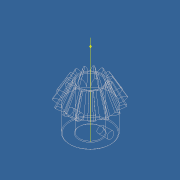
# Autodesk Inventor part: Bevel Gear2
Saved by Autodesk Inventor 2012 SP2 (Build 160219200, 219)
## iProperties
Created: 2012-07-24
Part Number: Bevel Gear2
Material: Steel, Mild
Document SubType Name: Modeling
Designer: bruno.silveira
Categories: <?xml version="1.0" encoding="UTF-16"?> <MemberInstance><Categories><FamilyTemplate><FamilyTemplateParameter ValueType="xs:double" Id="1" ObjectReferenceKey="da_z" ObjectType="kUserParameterObject"/><FamilyTemplateParameter ValueType="xs:double" Id="2" ObjectReferenceKey="da_b" ObjectType="kUserParameterObject"/><FamilyTemplateParameter ValueType="xs:double" Id="3" ObjectReferenceKey="da_beta" ObjectType="kUserParameterObject"/><FamilyTemplateParameter ValueType="xs:double" Id="4" ObjectReferenceKey="da_dae" ObjectType="kUserParameterObject"/><FamilyTemplateParameter ValueType="xs:double" Id="5" ObjectReferenceKey="da_ve" ObjectType="kUserParameterObject"/><FamilyTemplateParameter ValueType="xs:double" Id="6" ObjectReferenceKey="da_omega" ObjectType="kUserParameterObject"/><FamilyTemplateParameter ValueType="xs:string" Id="7" ObjectReferenceKey="EAIAABAAAAAAHwAAAAAAAIAAAAAAAAAA" ObjectType="83914240" SubObjectId="SurfaceGeometry"/></FamilyTemplate><ParamToTemplateMap><ParamToTemplate CategoryParameter="//CategoryParameter[@InternalName='046C89C9-8512-4d59-83FE-43B91F4F132A']" TemplateParameter="1"/><ParamToTemplate CategoryParameter="//CategoryParameter[@InternalName='2552DF32-E462-4b46-AEBF-C6C7768E72AC']" TemplateParameter="2"/><ParamToTemplate CategoryParameter="//CategoryParameter[@InternalName='C9EE641D-15FC-4fae-A226-E94C4372FDD7']" TemplateParameter="3"/><ParamToTemplate><ParamToTemplate CategoryParameter="//CategoryParameter[@InternalName='00B6519A-459B-49c7-AD84-2E56D39A5744']" ConstantValue="-0.000000"/></ParamToTemplate><ParamToTemplate><ParamToTemplate CategoryParameter="//CategoryParameter[@InternalName='04B31F0E-C7A6-4894-AA32-9629BEFACF47']" ConstantValue="1.000000"/></ParamToTemplate><ParamToTemplate><ParamToTemplate CategoryParameter="//CategoryParameter[@InternalName='43CBEC2E-7847-49e7-A936-2F7889FCB2D9']" ConstantValue="0.200000"/></ParamToTemplate><ParamToTemplate><ParamToTemplate CategoryParameter="//CategoryParameter[@InternalName='B1EFC894-105D-4ebd-86BF-FA20ED196853']" ConstantValue="0.300000"/></ParamToTemplate><ParamToTemplate><ParamToTemplate CategoryParameter="//CategoryParameter[@InternalName='51175063-3D10-4879-93E8-6246FE8B403D']" ConstantValue="2060000000.000000"/></ParamToTemplate><ParamToTemplate><ParamToTemplate CategoryParameter="//CategoryParameter[@InternalName='A3A52E27-4454-46a9-B0BD-C932399B70AF']" ConstantValue="0.300000"/></ParamToTemplate><ParamToTemplate CategoryParameter="//CategoryParameter[@InternalName='2A200944-5A8C-41ca-B96E-8520D2E510F1']" TemplateParameter="4"/><ParamToTemplate><ParamToTemplate CategoryParameter="//CategoryParameter[@InternalName='1A637F62-92C8-44bc-B81F-10802510B579']" ConstantValue="1.516492"/></ParamToTemplate><ParamToTemplate CategoryParameter="//CategoryParameter[@InternalName='B52DD4BE-6863-48fb-BF58-89EF6F9EC65C']" TemplateParameter="5"/><ParamToTemplate><ParamToTemplate CategoryParameter="//CategoryParameter[@InternalName='3956BFF2-84D2-457d-93C2-9B0613DEBA67']" ConstantValue="1.315343"/></ParamToTemplate><ParamToTemplate CategoryParameter="//CategoryParameter[@InternalName='739CFA02-461B-4bf8-8049-181FCAD8B28F']" TemplateParameter="6"/><ParamToTemplate><ParamToTemplate CategoryParameter="//CategoryParameter[@InternalName='A27E999F-E2CE-4481-8A2A-EBF499C4C3C5']" ConstantValue="-0.000000"/></ParamToTemplate><ParamToTemplate><ParamToTemplate CategoryParameter="//CategoryParameter[@InternalName='9E1B4470-B2D3-4ff1-B813-535BB4CDF51A']" ConstantValue="3520000.000000"/></ParamToTemplate><ParamToTemplate><ParamToTemplate CategoryParameter="//CategoryParameter[@InternalName='F8452263-BFF6-458c-9FB1-07C4B99E95CD']" ConstantValue="11400000.000000"/></ParamToTemplate><ParamToTemplate><ParamToTemplate CategoryParameter="//CategoryParameter[@InternalName='3E3BB259-FD49-497f-8171-6EBC954A3479']" ConstantValue="2.000000"/></ParamToTemplate><ParamToTemplate CategoryParameter="//CategoryParameter[@InternalName='27C3BAF2-7550-4e4b-AE2C-0DB134B7D9B7']" TemplateParameter="7"/></ParamToTemplateMap><Category DisplayName="Gear" InternalName="DC85795E-93AB-48d5-8EEE-5A27447B64BD" Mnemonic="Gear"><CategoryParameter DisplayName="z" InternalName="046C89C9-8512-4d59-83FE-43B91F4F132A" Mnemonic="z"/><CategoryParameter DisplayName="b" InternalName="2552DF32-E462-4b46-AEBF-C6C7768E72AC" Mnemonic="b"/><CategoryParameter DisplayName="||b|" InternalName="C9EE641D-15FC-4fae-A226-E94C4372FDD7" Mnemonic="beta"/><CategoryParameter DisplayName="x" InternalName="00B6519A-459B-49c7-AD84-2E56D39A5744" Mnemonic="x"/><CategoryParameter DisplayName="a*" InternalName="04B31F0E-C7A6-4894-AA32-9629BEFACF47" Mnemonic="a"/><CategoryParameter DisplayName="c*" InternalName="43CBEC2E-7847-49e7-A936-2F7889FCB2D9" Mnemonic="c"/><CategoryParameter DisplayName="r|.f|*" InternalName="B1EFC894-105D-4ebd-86BF-FA20ED196853" Mnemonic="rf"/><CategoryParameter DisplayName="E" InternalName="51175063-3D10-4879-93E8-6246FE8B403D" Mnemonic="E"/><CategoryParameter DisplayName="||m|" InternalName="A3A52E27-4454-46a9-B0BD-C932399B70AF" Mnemonic="mi"/><Category DisplayName="BevelGear" InternalName="0C98F69A-0C2B-4791-B2FE-7691BB227E77" Mnemonic="BevelGear"><CategoryParameter DisplayName="d|.ae|" InternalName="2A200944-5A8C-41ca-B96E-8520D2E510F1" Mnemonic="dae"/><CategoryParameter DisplayName="d|.ai|" InternalName="1A637F62-92C8-44bc-B81F-10802510B579" Mnemonic="dai"/><CategoryParameter DisplayName="A|.e|" InternalName="B52DD4BE-6863-48fb-BF58-89EF6F9EC65C" Mnemonic="ve"/><CategoryParameter DisplayName="A|.i|" InternalName="3956BFF2-84D2-457d-93C2-9B0613DEBA67" Mnemonic="vi"/><CategoryParameter DisplayName="||S|" InternalName="739CFA02-461B-4bf8-8049-181FCAD8B28F" Mnemonic="omega"/><CategoryParameter DisplayName="x|.t|" InternalName="A27E999F-E2CE-4481-8A2A-EBF499C4C3C5" Mnemonic="xt"/><CategoryParameter DisplayName="||s||.Flim|" InternalName="9E1B4470-B2D3-4ff1-B813-535BB4CDF51A" Mnemonic="sFlim"/><CategoryParameter DisplayName="||s||.Hlim|" InternalName="F8452263-BFF6-458c-9FB1-07C4B99E95CD" Mnemonic="sHlim"/><CategoryParameter DisplayName="type" InternalName="3E3BB259-FD49-497f-8171-6EBC954A3479" Mnemonic="type"/><CategoryParameter DisplayName="PitchDiameter" InternalName="27C3BAF2-7550-4e4b-AE2C-0DB134B7D9B7" Mnemonic="IDS_PITCHDIAM"/></Category></Category></Categories></MemberInstance>
Mass: 60.9118 g
Surface Area: 34.3074 cm^2
Volume: 7.7496 cm^3
Density: 7.86 g/cm^3
CustomPartVersion: 1
Author: bruno.silveira
Autodesk Inventor part; units mm, degrees
ref_plane "Mesh Plane2" through (0, 0, 0) normal (0.9781476, 0.2079117, 0) x (0, 0, 1)
sketch "Teeth Body Sketch" plane through (0, 0, 0) normal (1, 0, 0) x (0, 1, 0)
  line L0 (0, 0) -> (9.640031, -23.304984) construction
  line L1 (9.640031, -23.304984) -> (12.585483, -21.832259)
  line L2 (12.585483, -21.832259) -> (0, 0) construction
  line L3 (11.25, -22.5) -> (0, 0) construction
  line L4 (5.807895, -14.040713) -> (7.582462, -13.153429)
  line L5 (9.640031, -23.304984) -> (5.807895, -14.040713)
  line L6 (12.585483, -21.832259) -> (7.582462, -13.153429)
  line L7 (0, -39.386751) -> (0, 6.564458)
  line L8 (0, -22.5) -> (12.585483, -22.5) construction
  dimension "d0" = 22.5
  dimension "d1" = 19.28006
  dimension "d2" = 25.17097
  dimension "d3" = 10
  dimension "d4" = 21.83226
  constraints: 16 end point, 4 point on line, 3 perpendicular, 2 collinear, 1 horizontal alignment, 1 vertical alignment
  measures "d0" diameter of L3.start L7
  measures "d1" diameter of L0.end L7
  measures "d2" diameter of L1.end L7
  measures "d3" distance between parallel lines of L1 L4
  measures "d4" vertical distance of L1.end L0.start
revolve "Teeth Body" add sketch "Teeth Body Sketch" angle 360 about axis through (0, 0, 0) along (0, 0, 1)
ref_plane "Tooth Plane" through (0, 11.25, -22.5) normal (0, -0.4472136, 0.8944272) x (1, 0, 0)
sketch "Start Sketch" plane through (0, 11.25, -22.5) normal (0, -0.4472136, 0.8944272) x (1, 0, 0)
  line L0 (0, -23.505131) -> (0, 10.644758)
  arc A0 (-0.686149, -2.195174) -> (-3.356057, 2.102319) centre (-5.477944, -2.194063) ccw
  arc A1 (3.356057, 2.102319) -> (0.686149, -2.195174) centre (5.477944, -2.194063) ccw
  line L1 (-0.686149, -2.195174) -> (0.686149, -2.195174)
  arc A2 (3.356057, 2.102319) -> (-3.356057, 2.102319) centre (0, -12.577882) ccw
  dimension "d7" = 4.7918
  dimension "d8" = 5.47794
  dimension "d9" = 10.38382
  dimension "d57" = 15.05893
  dimension "d58" = 10.38271
  constraints: 6 point on circle, 3 centre point, 3 symmetric about line, 2 end point, 1 coincident, 1 perpendicular, 1 other
  measures "d7" radius of A0
  measures "d8" horizontal distance of point (0, -12.578) A0.centre
  measures "d9" vertical distance of point (0, -12.578) A0.centre
  measures "d57" radius of A2
  measures "d58" distance from line of A2.centre L1
sketch "End Sketch" plane through (0, 6.704228, -13.408455) normal (0, -0.4472136, 0.8944272) x (1, 0, 0)
  line L0 (0, -15.358918) -> (0, 6.982715)
  arc A0 (-0.409584, -1.29779) -> (-2.003336, 1.267518) centre (-3.269956, -1.297127) ccw
  arc A1 (2.003336, 1.267518) -> (0.409584, -1.29779) centre (3.269956, -1.297127) ccw
  line L1 (-0.409584, -1.29779) -> (0.409584, -1.29779)
  arc A2 (2.003336, 1.267518) -> (-2.003336, 1.267518) centre (0, -7.495554) ccw
  dimension "d12" = 2.86037
  dimension "d15" = 3.26996
  dimension "d16" = 6.19843
  dimension "d59" = 8.98915
  dimension "d60" = 6.19776
  constraints: 6 point on circle, 3 centre point, 3 symmetric about line, 2 end point, 1 coincident, 1 other
  measures "d12" radius of A0
  measures "d15" horizontal distance of A0.centre point (0, -7.496)
  measures "d16" vertical distance of A0.centre point (0, -7.496)
  measures "d59" radius of A2
  measures "d60" distance from line of A2.centre L1
loft "Loft" cut profiles "Start Sketch", "End Sketch"
pattern_circular "Circular Pattern" count 15 over 360 about axis through (0, 0, 0) along (0, 0, 1) of "Loft"
ref_plane "End Plane" through (0, 6.704228, -13.408455) normal (0, -0.4472136, 0.8944272) x (1, 0, 0)
sketch3d "3D Sketch Right"
ref_plane "End Plane Right" through (-2.675041, 6.147424, -13.408455) normal (0.1784419, -0.4100713, 0.8944272) x (0.9169474, 0.3990081, 0)
sketch "End Sketch Right" plane through (-2.675041, 6.147424, -13.408455) normal (0.1784419, -0.4100713, 0.8944272) x (0.9169474, 0.3990081, 0)
  arc A0 (-0.409584, -1.29779) -> (-2.003336, 1.267518) centre (-3.269956, -1.297127) ccw
  line L0 (0, -21.405112) -> (0, 13.028898)
  arc A1 (2.003336, 1.267518) -> (0.409584, -1.29779) centre (3.269956, -1.297127) ccw
  line L1 (-0.409584, -1.29779) -> (0.409584, -1.29779)
  arc A2 (2.003336, 1.267518) -> (-2.003336, 1.267518) centre (0, -7.495554) ccw
  dimension "d70" = 3.26996
  dimension "d71" = 6.19843
  dimension "d72" = 2.86037
  dimension "d73" = 6.19776
  dimension "d74" = 8.98915
  constraints: 6 point on circle, 3 centre point, 3 symmetric about line, 2 end point, 1 coincident, 1 perpendicular, 1 other
  measures "d70" horizontal distance of A2.centre A0.centre
  measures "d71" vertical distance of point (0, -7.496) A0.centre
  measures "d72" radius of A0
  measures "d73" distance from line of point (0, -7.496) L1
  measures "d74" radius of A2
feature "Loft Right" [suppressed]
pattern_circular "Circular Pattern Right" [suppressed]
sketch3d "3D Sketch Left"
ref_plane "End Plane Left" through (2.623677, 6.147424, -13.3935) normal (-0.1752782, -0.4106867, 0.8947703) x (0.9197363, -0.3925369, 0)
sketch "End Sketch Left" plane through (2.623677, 6.147424, -13.3935) normal (-0.1752782, -0.4106867, 0.8947703) x (0.9197363, -0.3925369, 0)
  line L0 (0, -37.602181) -> (0, 20.60385)
  arc A0 (-0.409584, -1.286276) -> (-2.003336, 1.279032) centre (-3.269956, -1.285613) ccw
  arc A1 (2.003336, 1.279032) -> (0.409584, -1.286276) centre (3.269956, -1.285613) ccw
  line L1 (-0.409584, -1.286276) -> (0.409584, -1.286276)
  ellipse E0 centre (0, -5.873357) end of major axis (7.582462, -5.873357) minor radius 6.784562
  arc A2 (2.003336, 1.279032) -> (-2.003336, 1.279032) centre (0, -7.484041) ccw
  dimension "d56" = 6.78456
  dimension "d30" = 2.86037
  dimension "d31" = 3.26996
  dimension "d32" = 6.19843
  dimension "d61" = 8.98915
  dimension "d62" = 6.19776
  constraints: 6 point on circle, 3 centre point, 3 symmetric about line, 2 end point, 1 coincident, 2 other
  measures "d30" radius of A0
  measures "d31" horizontal distance of point (0, -7.484) A0.centre
  measures "d32" vertical distance of A0.centre point (0, -7.484)
  measures "d61" radius of A2
  measures "d62" distance from line of point (0, -7.484) L1
feature "Loft Left" [suppressed]
pattern_circular "Circular Pattern Left" [suppressed]
sketch "Body Sketch" plane through (0, 0, 0) normal (1, 0, 0) x (0, 1, 0)
  line L0 (0, -35.037536) -> (0, -19.530831)
  line L1 (9.640031, -23.304984) -> (5.807895, -14.040713)
  line L2 (5.807895, -14.040713) -> (0, -14.040713)
  line L3 (9.640031, -23.304984) -> (0, -23.304984)
  constraints: 4 end point, 2 perpendicular, 2 point on line
sketch "Body Sketch outline for Fix Body" plane through (0, 0, 0) normal (1, 0, 0) x (0, 1, 0)
  line L0 (0, -23.304984) -> (9.640031, -23.304984)
  line L1 (0, -14.040713) -> (0, -23.304984)
  line L2 (5.807895, -14.040713) -> (0, -14.040713)
  line L3 (9.640031, -23.304984) -> (5.807895, -14.040713)
revolve "Fix Body" add sketch "Body Sketch outline for Fix Body" angle 360 about axis through (0, 0, 0) along (0, 0, 1)
sketch "Sketch6" plane through (0, 0, 0) normal (1, 0, 0) x (0, 1, 0)
  line L0 (11.25, -22.5) -> (0, 0)
  line L1 (0, -37.799919) -> (0, 6.299986)
surface revolve "Pitch Diameter" sketch "Sketch6" angle 360 about axis through (0, 0, 0) along (0, 0, 1) shown no curves L0
sketch "Sketch8" plane through (0, 0, -23.304984) normal (0, 0, -1) x (-1, 0, 0)
  arc A0 (0.700173, 9.61457) -> (-0.700173, 9.61457) centre (0, 0) ccw
  arc A1 (-0.700173, 9.61457) -> (-3.270958, 9.068133) centre (0, 0) ccw
  arc A2 (-3.270958, 9.068133) -> (-4.550238, 8.498561) centre (0, 0) ccw
  arc A3 (-4.550238, 8.498561) -> (-6.676511, 6.953733) centre (0, 0) ccw
  arc A4 (-6.676511, 6.953733) -> (-7.613525, 5.913073) centre (0, 0) ccw
  arc A5 (-7.613525, 5.913073) -> (-8.927634, 3.63697) centre (0, 0) ccw
  arc A6 (-8.927634, 3.63697) -> (-9.360365, 2.305161) centre (0, 0) ccw
  arc A7 (-9.360365, 2.305161) -> (-9.635088, -0.308658) centre (0, 0) ccw
  arc A8 (-9.635088, -0.308658) -> (-9.488712, -1.701334) centre (0, 0) ccw
  arc A9 (-9.488712, -1.701334) -> (-8.676549, -4.200917) centre (0, 0) ccw
  arc A10 (-8.676549, -4.200917) -> (-7.976375, -5.413653) centre (0, 0) ccw
  arc A11 (-7.976375, -5.413653) -> (-6.217755, -7.366799) centre (0, 0) ccw
  arc A12 (-6.217755, -7.366799) -> (-5.08485, -8.189902) centre (0, 0) ccw
  arc A13 (-5.08485, -8.189902) -> (-2.683854, -9.258894) centre (0, 0) ccw
  arc A14 (-2.683854, -9.258894) -> (-1.314109, -9.550043) centre (0, 0) ccw
  arc A15 (-1.314109, -9.550043) -> (1.314109, -9.550043) centre (0, 0) ccw
  arc A16 (1.314109, -9.550043) -> (2.683854, -9.258894) centre (0, 0) ccw
  arc A17 (2.683854, -9.258894) -> (5.08485, -8.189902) centre (0, 0) ccw
  arc A18 (5.08485, -8.189902) -> (6.217755, -7.366799) centre (0, 0) ccw
  arc A19 (6.217755, -7.366799) -> (7.976375, -5.413653) centre (0, 0) ccw
  arc A20 (7.976375, -5.413653) -> (8.676549, -4.200917) centre (0, 0) ccw
  arc A21 (8.676549, -4.200917) -> (9.488712, -1.701334) centre (0, 0) ccw
  arc A22 (9.488712, -1.701334) -> (9.635088, -0.308658) centre (0, 0) ccw
  arc A23 (9.635088, -0.308658) -> (9.360365, 2.305161) centre (0, 0) ccw
  arc A24 (9.360365, 2.305161) -> (8.927634, 3.63697) centre (0, 0) ccw
  arc A25 (8.927634, 3.63697) -> (7.613525, 5.913073) centre (0, 0) ccw
  arc A26 (7.613525, 5.913073) -> (6.676511, 6.953733) centre (0, 0) ccw
  arc A27 (6.676511, 6.953733) -> (4.550238, 8.498561) centre (0, 0) ccw
  arc A28 (4.550238, 8.498561) -> (3.270958, 9.068133) centre (0, 0) ccw
  arc A29 (3.270958, 9.068133) -> (0.700173, 9.61457) centre (0, 0) ccw
  circle A30 centre (0, 0) radius 9
  dimension "d94" = 18
  constraints: 1 centre point, 1 coincident
  measures "d94" diameter of A30
extrude "Extrusion1" add sketch "Sketch8" along normal blind 11.7 contours A29 A28 A27 A26 A25 A24 A23 A22 A21 A20 A19 A18 A17 A16 A15 A14 A13 A12 A11 A10 A9 A8 A7 A6 A5 A4 A3 A2 A1 A0 | A30
sketch "Sketch9" plane through (0, 0, -35.004984) normal (0, 0, -1) x (-1, 0, 0)
  circle A0 centre (0, 0) radius 9.640031
  circle A1 centre (0, 0) radius 5
  dimension "d97" = 10
  constraints: 1 centre point, 1 coincident
  measures "d97" diameter of A1
extrude "Extrusion2" cut sketch "Sketch9" against normal blind 25 contours A1
chamfer "Chamfer1" distance 0.3 angle 45 3 edges at (-2.6839, 9.2589, -35.005) (5, 0, -35.005) (5, 0, -14.0407)
sketch "Sketch10" plane through (0, 0, 0) normal (1, 0, 0) x (0, 1, 0)
  circle A0 centre (0, -31.004984) radius 1.5875
  line L0 (9.340031, -35.004984) -> (-9.340031, -35.004984)
  point P0 (0, 0)
  dimension "d103" = 3.175
  dimension "d104" = 4
  constraints: 1 centre point
  measures "d103" diameter of A0
  measures "d104" distance from line of L0 A0.centre
extrude "Extrusion3" cut sketch "Sketch10" along normal mid plane 20
equation "\"d0\" = da_de"
equation "\"d1\" = da_dfe"
equation "\"d2\" = da_dae"
equation "\"d3\" = da_b"
equation "\"d4\" = da_ve"
equation "\"d7\" = fd_rr"
equation "\"d8\" = fd_x"
equation "\"d9\" = fd_y"
equation "\"d57\" = 0.5 * fd_dva + 0.3 * da_he"
equation "\"d58\" = 0.5 * fd_dva - 1.12 * da_he"
equation "\"da_teethtype\" = 0"
equation "\"da_b\" = 10"
equation "\"da_de\" = 22.5"
equation "\"da_dae\" = 25.17097"
equation "\"da_dfe\" = 19.28006"
equation "\"da_le\" = 25.15576"
equation "\"da_omega\" = 90deg"
equation "\"da_beta\" = 0"
equation "\"da_delta\" = 26.565051deg"
equation "\"da_alpha\" = 20deg"
equation "\"da_he\" = 3.29312"
equation "\"da_ve\" = 21.83226"
equation "\"da_zv\" = 16.77051"
equation "\"fd_loft\" = da_b + 0.05 * da_he"
equation "\"fd_x\" = fd_x1 + fd_x2"
equation "\"fd_y\" = fd_y1 - fd_y2"
equation "\"fd_dd\" = fd_dva - 0.8 * da_he"
equation "\"da_dvw\" = 25.15576"
equation "\"d11\" = fd_loft"
equation "\"da_dm\" = 18.02786"
equation "\"da_x\" = 0"
equation "\"da_m\" = 1.5"
equation "\"d50\" = da_omega"
equation "\"fd_rr\" = 4.791795"
equation "\"fd_dva\" = 28.141995"
equation "\"fd_x1\" = 1.189407"
equation "\"fd_x2\" = 4.288537"
equation "\"fd_y1\" = 12.521519"
equation "\"fd_y2\" = 2.137699"
body "Solid1"
body "Srf1"
